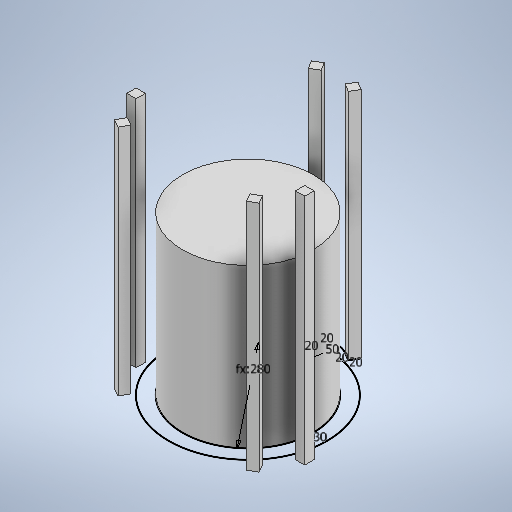
# Autodesk Inventor part: RT_FRM_SK_001_RoughDim
Saved by Autodesk Inventor 2025.3 (Build 293356000, 356)
## iProperties
Created: 2026-04-19
Part Number: RT_FRM_SK_001_RoughDim
Material: Generic
Document SubType Name: Modeling
Designer: louis
Density: 1 g/cm^3
Appearance: Default
Author: louis
Autodesk Inventor part; units mm, degrees
ref_plane "YZ Plane" through (0, 0, 0) normal (1, 0, 0) x (0, 1, 0)
ref_plane "XZ Plane" through (0, 0, 0) normal (0, 1, 0) x (-1, 0, 0)
ref_plane "XY Plane" through (0, 0, 0) normal (0, 0, 1) x (1, 0, 0)
sketch "Sketch1" plane through (0, 0, 0) normal (0, 1, 0) x (-1, 0, 0)
  circle A0 centre (0, 0) radius 140
  line L0 (53.1984, -189.6984) -> (36.0555, -200)
  line L1 (36.0555, -200) -> (25.7539, -182.8571)
  line L2 (25.7539, -182.8571) -> (42.8968, -172.5556)
  line L3 (42.8968, -172.5556) -> (53.1984, -189.6984)
  circle A1 centre (0, 0) radius 170
  arc A2 (-25.7539, -182.8571) -> (25.7539, -182.8571) centre (0, -140) ccw
  line L4 (0, 0) -> (0, -140) construction
  line L5 (-36.0555, -200) -> (-53.1984, -189.6984)
  line L6 (-53.1984, -189.6984) -> (-42.8968, -172.5556)
  line L7 (-42.8968, -172.5556) -> (-25.7539, -182.8571)
  line L8 (-25.7539, -182.8571) -> (-36.0555, -200)
  dimension "d0" = 280
  dimension "d3" = 20
  dimension "d5" = 20
  dimension "d6" = 30
  dimension "d7" = 20
  dimension "d8" = 20
  dimension "d9" = 50
  constraints: 18 end point, 4 parallel, 4 tangent, 2 centre point, 2 coincident, 2 perpendicular, 2 point on circle, 1 symmetric about line, 1 vertical, 1 vertical alignment, 2 other
  measures "d3" distance of L1.end L2.end
  measures "d5" distance of L0.end L1.end
  measures "d7" distance of L7.end L6.end
  measures "d8" distance of L5.end L6.end
  measures "d9" radius of A2
extrude "Extrusion1" add sketch "Sketch1" along normal blind 340 contours A0
extrude "Extrusion2" add sketch "Sketch1" along normal blind 500 contours L0 L1 L2 L3 | L5 L6 L7 L8
pattern_circular "Circular Pattern1" count 3 over 360 about axis through (0, 0, 0) along (0, 1, 0) of "Extrusion2"
equation "\"d0\" = 2 * Rmax"
equation "\"d1\" = Zmin"
equation "\"d10\" = Hmax"
equation "\"Zmin\" = 340"
equation "\"Hmax\" = 500"
equation "\"Rmax\" = 140"
body "Solid1"
